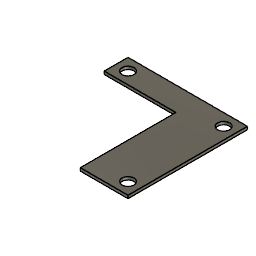
WeldingRobot_BracketAssembly (Autodesk Fusion 360 archive; units mm, degrees)
design "Base_Plate"
Autodesk Fusion 360 part; units mm, degrees
sketch "Sketch1" plane through (0, 0, 0) normal (0, 0, 1) x (1, 0, 0)
  line L0 (152.4, 0) -> (254, 0)
  line L1 (254, 0) -> (254, 254)
  line L2 (254, 254) -> (0, 254)
  line L3 (0, 254) -> (0, 203.2)
  line L4 (152.4, 0) -> (152.4, 203.2)
  line L5 (152.4, 203.2) -> (0, 203.2)
  dimension "d1" = 254
  dimension "d2" = 254
  dimension "d3" = 152.4
  dimension "d4" = 203.2
  constraint horizontal L0
  constraint vertical L1
  constraint horizontal L2
  constraint vertical L3
  constraint vertical L4
  constraint horizontal L5
  measures "d1" distance of origin L0.end
  measures "d2" distance of origin L2.end
  measures "d3" distance of origin L0.start
  measures "d4" distance of origin L3.end
extrude "Extrude1" add sketch "Sketch1" along normal blind 6.35
sketch "Sketch2" plane through (0, 0, 6.35) normal (0, 0, 1) x (-1, 0, 0)
  line L0 (-152.4, 0) -> (-254, 0)
  line L1 (-254, 0) -> (-254, -254)
  line L2 (-254, -254) -> (0, -254)
  line L3 (0, -254) -> (0, -203.2)
  line L4 (0, -203.2) -> (-152.4, -203.2)
  line L5 (-152.4, -203.2) -> (-152.4, 0)
  circle A0 centre (-228.6, -25.4) radius 12.7
  circle A1 centre (-228.6, -228.6) radius 12.7
  circle A2 centre (-25.4, -228.6) radius 12.7
  dimension "d7" = 25.4
  dimension "d8" = 25.4
  dimension "d9" = 25.4
  measures "d7" diameter of A0
  measures "d8" diameter of A1
  measures "d9" diameter of A2
extrude "Extrude2" cut sketch "Sketch2" against normal blind 25.4 contours A0 | A1 | A2

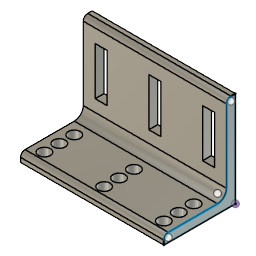
design "Steel_Bracket"
Autodesk Fusion 360 part; units mm, degrees
sketch "Sketch1" plane through (0, 0, 0) normal (0, 1, 0) x (1, 0, 0)
  line L0 (0, 0) -> (-152.4, 0)
  line L1 (-152.4, 0) -> (-152.4, -9.525)
  line L2 (-9.525, -203.2) -> (0, -203.2)
  line L3 (0, -203.2) -> (0, 0)
  line L4 (0, -203.2) -> (-9.525, -203.2)
  line L5 (-152.4, 0) -> (-152.4, -9.525)
  line L6 (-142.875, -19.05) -> (-38.1, -19.05)
  line L7 (-142.875, -19.05) -> (-38.1, -19.05)
  line L8 (-19.05, -38.1) -> (-19.05, -193.675)
  arc A0 (-19.05, -193.675) -> (-9.525, -203.2) centre (-9.525, -193.675) ccw
  arc A1 (-152.4, -9.525) -> (-142.875, -19.05) centre (-142.875, -9.525) ccw
  arc A2 (-19.05, -38.1) -> (-38.1, -19.05) centre (-38.1, -38.1) ccw
  dimension "d3" = 9.525
  dimension "d4" = 9.525
  dimension "d5" = 19.05
  dimension "WIDTH" = 152.4
  dimension "HEIGHT" = 203.2
  constraint horizontal L0
  constraint vertical L1
  constraint horizontal L2
  constraint vertical L3
  constraint coincident L0.start L3.end
  constraint perpendicular L3 L4
  constraint perpendicular L0 L5
  constraint perpendicular L5 L6
  constraint perpendicular L5 L7
  constraint perpendicular L2 L8
  constraint tangent L2 A0
  constraint tangent L8 A0
  constraint tangent L5 A1
  constraint tangent L7 A1
  constraint tangent L7 A2
  constraint tangent L8 A2
  measures "d3" radius of A0
  measures "d4" radius of A1
  measures "d5" radius of A2
  measures "WIDTH" distance of L0.start L0.end
  measures "HEIGHT" distance of L0.start L2.end
extrude "Extrude1" add sketch "Sketch1" along normal blind 304.8
sketch "Sketch2" plane through (0, 0, 19.05) normal (0, 0, 1) x (-1, 0, 0)
  line L0 (142.875, 0) -> (38.1, 0)
  line L1 (38.1, 0) -> (38.1, -304.8)
  line L2 (38.1, -304.8) -> (142.875, -304.8)
  line L3 (142.875, -304.8) -> (142.875, 0)
  circle A0 centre (127, -25.4) radius 12.7
  circle A1 centre (95.25, -25.4) radius 12.7
  circle A2 centre (63.5, -25.4) radius 12.7
  circle A3 centre (127, -152.4) radius 12.7
  circle A4 centre (95.25, -152.4) radius 12.7
  circle A5 centre (63.5, -152.4) radius 12.7
  circle A6 centre (127, -279.4) radius 12.7
  circle A7 centre (95.25, -279.4) radius 12.7
  circle A8 centre (63.5, -279.4) radius 12.7
  dimension "d12" = -63.5
  dimension "d13" = -254
extrude "Extrude2" cut sketch "Sketch2" against normal blind 50.8 contours A0 | A1 | A2 | A3 | A4 | A5 | A6 | A7 | A8
sketch "Sketch3" plane through (-19.05, 0, 0) normal (-1, 0, 0) x (0, -1, 0)
  line L0 (0, 38.1) -> (0, 193.675)
  line L1 (0, 193.675) -> (-304.8, 193.675)
  line L2 (-304.8, 193.675) -> (-304.8, 38.1)
  line L3 (-304.8, 38.1) -> (0, 38.1)
  line L4 (-279.4, 165.1) -> (-254, 165.1)
  line L5 (-254, 165.1) -> (-254, 63.5)
  line L6 (-254, 63.5) -> (-279.4, 63.5)
  line L7 (-279.4, 63.5) -> (-279.4, 165.1)
  line L8 (-139.7, 165.1) -> (-139.7, 63.5)
  line L9 (-165.1, 63.5) -> (-165.1, 165.1)
  line L10 (-139.7, 63.5) -> (-165.1, 63.5)
  line L11 (-165.1, 165.1) -> (-139.7, 165.1)
  line L12 (-25.4, 165.1) -> (-25.4, 63.5)
  line L13 (-50.8, 63.5) -> (-50.8, 165.1)
  line L14 (-25.4, 63.5) -> (-50.8, 63.5)
  line L15 (-50.8, 165.1) -> (-25.4, 165.1)
  dimension "d18" = 228.6
  dimension "d19" = 0
  constraint horizontal L4
  constraint vertical L5
  constraint horizontal L6
  constraint vertical L7
extrude "Extrude3" cut sketch "Sketch3" against normal blind 76.2 contours L4 L5 L6 L7 | L8 L9 L10 L11 | L12 L13 L14 L15
